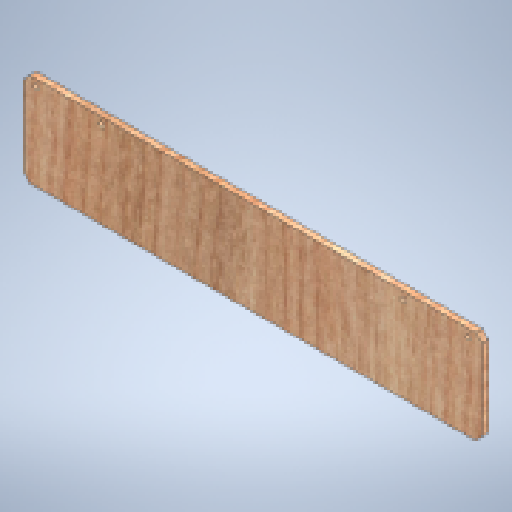
# Autodesk Inventor part: фанера_электр
Saved by Autodesk Inventor 2023.1 (Build 271208000, 208)
## iProperties
Created: 2025-12-30
Part Number: фанера_электр
Material: Древесина (береза)
Document SubType Name: Modeling
Designer: DELL
Density: 0.55 g/cm^3
Appearance: Береза — натуральный — полированный
Author: DELL
Autodesk Inventor part; units mm, degrees
ref_plane "YZ Plane" through (0, 0, 0) normal (1, 0, 0) x (0, 1, 0)
ref_plane "XZ Plane" through (0, 0, 0) normal (0, 1, 0) x (-1, 0, 0)
ref_plane "XY Plane" through (0, 0, 0) normal (0, 0, 1) x (1, 0, 0)
sketch "Эскиз1" plane through (0, 0, 0) normal (0, 0, 1) x (1, 0, 0)
  line L0 (-16.3474, 23.4) -> (16.3474, 23.4) projected
  line L1 (250.5, 57.3225) -> (250.5, -9.6775) projected
  line L2 (236.5474, 23.3225) -> (203.8526, 23.3225) projected
  line L3 (-38.764, -20.3083) -> (241.736, -20.3083)
  line L4 (241.736, -20.3083) -> (241.736, 29.6917)
  line L5 (241.736, 29.6917) -> (-38.764, 29.6917)
  line L6 (-38.764, 29.6917) -> (-38.764, -20.3083)
  line L7 (-38.764, -20.3083) -> (241.736, 29.6917) construction
  line L8 (241.736, -20.3083) -> (-38.764, 29.6917) construction
  point P0 (101.486, 4.6917)
  dimension "d13" = 280.5
  dimension "d14" = 50
  constraints: 12 end point, 2 midpoint, 2 parallel, 1 horizontal, 1 perpendicular
  measures "d13" distance of L5.end L4.end
  measures "d14" distance of L4.end L3.end
extrude "Выдавливание1" add sketch "Эскиз1" along normal blind 4
